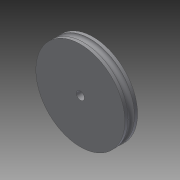
# Autodesk Inventor part: Pulley
Saved by Autodesk Inventor 2014 SP1 (Build 180222100, 222)
## iProperties
Created: 2014-01-27
Part Number: Pulley
Material: Generic
Document SubType Name: Modeling
Designer: tom
Density: 1 g/cm^3
Appearance: Default
Author: tom
Autodesk Inventor part; units mm, degrees
ref_plane "YZ Plane" through (0, 0, 0) normal (1, 0, 0) x (0, 1, 0)
ref_plane "XZ Plane" through (0, 0, 0) normal (0, 1, 0) x (-1, 0, 0)
ref_plane "XY Plane" through (0, 0, 0) normal (0, 0, 1) x (1, 0, 0)
sketch "Sketch1" plane through (0, 0, 0) normal (0, 0, 1) x (1, 0, 0)
  circle A0 centre (0, 0) radius 2.875
  circle A1 centre (0, 0) radius 4.875
  circle A2 centre (0, 0) radius 13.97
  dimension "d0" = 5.75
  dimension "d2" = 2
  dimension "d3" = 27.94
  constraints: 3 centre point, 2 coincident
  measures "d0" diameter of A0
  measures "d2" radial gap between concentric circles of A0 A1
  measures "d3" diameter of A2
extrude "Extrusion1" add sketch "Sketch1" against normal blind 4.064 contours A1
sketch "Sketch2" plane through (0, 0, 0) normal (0, 0, 1) x (1, 0, 0)
  circle A0 centre (0, 0) radius 4.875 projected
  circle A1 centre (0, 0) radius 1.27
  circle A2 centre (0, 0) radius 13.97
  dimension "d6" = 2.54
  dimension "d7" = 27.94
  constraints: 2 centre point, 2 coincident
  measures "d6" diameter of A1
  measures "d7" diameter of A2
extrude "Extrusion2" add sketch "Sketch2" along normal mid plane 4 contours A0 | A2
sketch "Sketch3" plane through (0, 0, 0) normal (1, 0, 0) x (0, 1, 0)
  line L0 (13.97, 2) -> (-13.97, 2) projected
  line L1 (-13.97, -2) -> (13.97, -2) projected
  line L2 (13.97, 2) -> (13.97, -2)
  circle A0 centre (13.97, 0) radius 1
  line L3 (0, 2) -> (0, -2) construction
  point P0 (0, 0)
  dimension "d10" = 2
  constraints: 4 end point, 3 midpoint, 1 centre point, 1 perpendicular
  measures "d10" diameter of A0
revolve "Revolution1" cut sketch "Sketch3" angle 360 about axis through (0, 0, 2) along (0, 0, -1)
sketch "Sketch4" plane through (0, 0, 2) normal (0, 0, 1) x (1, 0, 0)
  circle A0 centre (0, 0) radius 13.97 projected
  line L0 (0, 4.875) -> (0, 13.97)
  line L1 (0, 0) -> (9.9312, 0) construction
  circle A1 centre (-2.0844, -9.8063) radius 1
  arc A2 (0, 4.875) -> (-2.0603, -4.4183) centre (0, 0) ccw
  line L2 (-2.0603, -4.4183) -> (-5.904, -12.6611)
  dimension "d13" = 2
  constraints: 6 end point, 4 point on circle, 2 centre point, 1 coincident, 1 horizontal, 1 vertical
  measures "d13" diameter of A1
extrude "Extrusion3" cut sketch "Sketch4" against normal blind 4 contours L0 A2 L2 A0 | A1 picked at (-8.1024, 7.2275)
fillet "Fillet1" radius 3.175 2 edges at (0, 4.875, 0) (-2.0603, -4.4183, 0)
body "Solid1"
